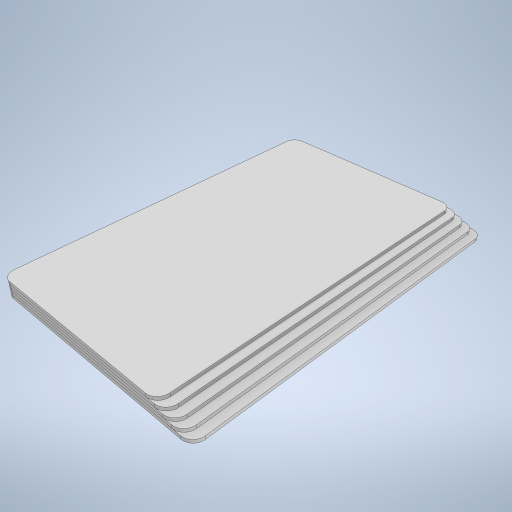
# Autodesk Inventor part: frame
Saved by Autodesk Inventor 2024 (Build 280153000, 153)
## iProperties
Created: 2023-10-17
Part Number: frame
Material: 常规
Document SubType Name: Modeling
Designer: Administrator
Density: 1 g/cm^3
Appearance: 默认
Author: Administrator
Autodesk Inventor part; units mm, degrees
ref_plane "YZ Plane" through (0, 0, 0) normal (1, 0, 0) x (0, 1, 0)
ref_plane "XY Plane" through (0, 0, 0) normal (0, 0, 1) x (1, 0, 0)
ref_plane "底层" through (0, -3, 0) normal (0, 1, 0) x (-1, 0, 0)
ref_plane "第二层" through (0, 3, 0) normal (0, 1, 0) x (-1, 0, 0)
ref_plane "第三层" through (0, 6, 0) normal (0, 1, 0) x (-1, 0, 0)
ref_plane "第四层" through (0, 9, 0) normal (0, 1, 0) x (-1, 0, 0)
ref_plane "第五层" through (0, 12, 0) normal (0, 1, 0) x (-1, 0, 0)
sketch "底层草图" plane through (0, -3, 0) normal (0, 1, 0) x (-1, 0, 0)
  line L0 (-97, 140) -> (-97, -140)
  arc A0 (-97, -140) -> (-90, -147) centre (-90, -140) ccw
  line L1 (-90, -147) -> (90, -147)
  arc A1 (90, -147) -> (97, -140) centre (90, -140) ccw
  line L2 (97, -140) -> (97, 140)
  arc A2 (97, 140) -> (90, 147) centre (90, 140) ccw
  line L3 (90, 147) -> (-90, 147)
  arc A3 (-90, 147) -> (-97, 140) centre (-90, 140) ccw
  point P0 (0, 0)
  constraints: 8 end point, 8 point on circle, 4 centre point
sketch "第一层草图" plane through (0, 0, 0) normal (0, 1, 0) x (-1, 0, 0)
  line L0 (90, 150) -> (-90, 150)
  line L1 (-100, 140) -> (-100, -140)
  line L2 (-90, -150) -> (90, -150)
  line L3 (100, -140) -> (100, 140)
  line L4 (100, 150) -> (-100, -150) construction
  line L5 (-100, 150) -> (100, -150) construction
  arc A0 (100, 140) -> (90, 150) centre (90, 140) ccw
  arc A1 (-90, 150) -> (-100, 140) centre (-90, 140) ccw
  arc A2 (-100, -140) -> (-90, -150) centre (-90, -140) ccw
  arc A3 (90, -150) -> (100, -140) centre (90, -140) ccw
  point P0 (0, 0)
  dimension "d2" = 200
  dimension "d3" = 300
  dimension "d4" = 10
  constraints: 12 end point, 8 point on circle, 8 point on line, 8 tangent, 4 centre point, 3 equal radius, 2 midpoint, 2 parallel, 1 horizontal, 1 perpendicular
  measures "d2" distance of L5.end L4.end
  measures "d3" distance of L4.end L5.start
  measures "d4" radius of A0
sketch "第二层草图" plane through (0, 3, 0) normal (0, 1, 0) x (-1, 0, 0)
  line L0 (100, -140) -> (100, 140) projected
  line L1 (100, 0) -> (-92.5, 0)
  line L2 (90, 150) -> (-82.5, 150)
  line L3 (-92.5, 140) -> (-92.5, -140)
  line L4 (-82.5, -150) -> (90, -150)
  line L5 (100, -140) -> (100, 140)
  line L6 (100, 150) -> (-92.5, -150) construction
  line L7 (-92.5, 150) -> (100, -150) construction
  arc A0 (100, 140) -> (90, 150) centre (90, 140) ccw
  arc A1 (-82.5, 150) -> (-92.5, 140) centre (-82.5, 140) ccw
  arc A2 (-92.5, -140) -> (-82.5, -150) centre (-82.5, -140) ccw
  arc A3 (90, -150) -> (100, -140) centre (90, -140) ccw
  point P0 (0, 0)
  point P1 (3.75, 0)
  dimension "d13" = 192.5
  dimension "d14" = 192.5
  dimension "d15" = 300
  dimension "d16" = 10
  constraints: 14 end point, 8 point on circle, 8 point on line, 8 tangent, 4 centre point, 4 midpoint, 3 equal radius, 2 horizontal, 2 parallel, 1 perpendicular
  measures "d13" distance of L1.start L1.end
  measures "d14" distance of L7.end L6.end
  measures "d15" distance of L6.end L7.start
  measures "d16" radius of A0
sketch "第三层草图" plane through (0, 6, 0) normal (0, 1, 0) x (-1, 0, 0)
  line L0 (100, -140) -> (100, 140) projected
  line L1 (100, 0) -> (-85, 0)
  line L2 (90, 150) -> (-75, 150)
  line L3 (-85, 140) -> (-85, -140)
  line L4 (-75, -150) -> (90, -150)
  line L5 (100, -140) -> (100, 140)
  line L6 (100, 150) -> (-85, -150) construction
  line L7 (-85, 150) -> (100, -150) construction
  arc A0 (100, 140) -> (90, 150) centre (90, 140) ccw
  arc A1 (-75, 150) -> (-85, 140) centre (-75, 140) ccw
  arc A2 (-85, -140) -> (-75, -150) centre (-75, -140) ccw
  arc A3 (90, -150) -> (100, -140) centre (90, -140) ccw
  point P0 (0, 0)
  point P1 (7.5, 0)
  dimension "d17" = 185
  dimension "d18" = 185
  dimension "d19" = 300
  dimension "d20" = 10
  constraints: 14 end point, 8 point on circle, 8 point on line, 8 tangent, 4 centre point, 4 midpoint, 3 equal radius, 2 horizontal, 2 parallel, 1 perpendicular
  measures "d17" distance of L1.start L1.end
  measures "d18" distance of L7.end L6.end
  measures "d19" distance of L6.end L7.start
  measures "d20" radius of A0
sketch "第四层草图" plane through (0, 9, 0) normal (0, 1, 0) x (-1, 0, 0)
  line L0 (100, -140) -> (100, 140) projected
  line L1 (100, 0) -> (-77.5, 0)
  line L2 (90, 150) -> (-67.5, 150)
  line L3 (-77.5, 140) -> (-77.5, -140)
  line L4 (-67.5, -150) -> (90, -150)
  line L5 (100, -140) -> (100, 140)
  line L6 (100, 150) -> (-77.5, -150) construction
  line L7 (-77.5, 150) -> (100, -150) construction
  arc A0 (100, 140) -> (90, 150) centre (90, 140) ccw
  arc A1 (-67.5, 150) -> (-77.5, 140) centre (-67.5, 140) ccw
  arc A2 (-77.5, -140) -> (-67.5, -150) centre (-67.5, -140) ccw
  arc A3 (90, -150) -> (100, -140) centre (90, -140) ccw
  point P0 (0, 0)
  point P1 (11.25, 0)
  dimension "d22" = 177.5
  dimension "d23" = 177.5
  dimension "d24" = 300
  dimension "d25" = 10
  constraints: 14 end point, 8 point on circle, 8 point on line, 8 tangent, 4 centre point, 4 midpoint, 3 equal radius, 2 horizontal, 2 parallel, 1 perpendicular
  measures "d22" distance of L1.start L1.end
  measures "d23" distance of L7.end L6.end
  measures "d24" distance of L6.end L7.start
  measures "d25" radius of A0
sketch "第五层草图" plane through (0, 12, 0) normal (0, 1, 0) x (-1, 0, 0)
  line L0 (100, -140) -> (100, 140) projected
  line L1 (100, 0) -> (-70, 0)
  line L2 (90, 150) -> (-60, 150)
  line L3 (-70, 140) -> (-70, -140)
  line L4 (-60, -150) -> (90, -150)
  line L5 (100, -140) -> (100, 140)
  line L6 (100, 150) -> (-70, -150) construction
  line L7 (-70, 150) -> (100, -150) construction
  arc A0 (100, 140) -> (90, 150) centre (90, 140) ccw
  arc A1 (-60, 150) -> (-70, 140) centre (-60, 140) ccw
  arc A2 (90, -150) -> (100, -140) centre (90, -140) ccw
  arc A3 (-70, -140) -> (-60, -150) centre (-60, -140) ccw
  point P0 (0, 0)
  point P1 (15, 0)
  dimension "d63" = 170
  dimension "d64" = 170
  dimension "d65" = 300
  dimension "d66" = 10
  constraints: 14 end point, 8 point on circle, 8 point on line, 8 tangent, 4 centre point, 4 midpoint, 3 equal radius, 2 horizontal, 2 parallel, 1 perpendicular
  measures "d63" distance of L1.start L1.end
  measures "d64" distance of L7.end L6.end
  measures "d65" distance of L6.end L7.start
  measures "d66" radius of A0
extrude "拉伸14" add sketch "底层草图" against normal blind 2
extrude "拉伸15" add sketch "第一层草图" against normal blind 3 separate body
extrude "拉伸16" add sketch "第二层草图" against normal blind 3 separate body
extrude "拉伸17" add sketch "第三层草图" against normal blind 3 separate body
extrude "拉伸18" add sketch "第四层草图" against normal blind 3 separate body
extrude "拉伸19" add sketch "第五层草图" against normal blind 3 separate body
